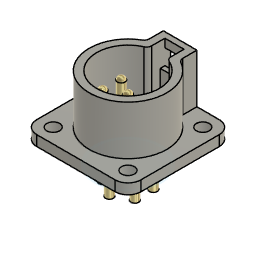
RPC1-12RB-6P_v13 (Autodesk Fusion 360 design; units mm, degrees)
Autodesk Fusion 360 part; units mm, degrees
sketch "Skizze1" plane through (0, 0, 0) normal (0, 0, 1) x (1, 0, 0)
  line L0 (-10.1, 10.1) -> (10.1, 10.1)
  line L1 (10.1, 10.1) -> (10.1, -10.1)
  line L2 (10.1, -10.1) -> (-10.1, -10.1)
  line L3 (-10.1, -10.1) -> (-10.1, 10.1)
  line L4 (0, 10.1) -> (0, -10.1) construction
  line L5 (-10.1, 0) -> (10.1, 0) construction
  line L6 (-7.25, 7.25) -> (7.25, 7.25) construction
  line L7 (7.25, 7.25) -> (7.25, -7.25) construction
  line L8 (7.25, -7.25) -> (-7.25, -7.25) construction
  line L9 (-7.25, -7.25) -> (-7.25, 7.25) construction
  circle A0 centre (0, 0) radius 7.5
  circle A1 centre (0, 0) radius 6.05
  line L10 (-3.25, 10.1) -> (3.25, 10.1)
  line L11 (3.25, 10.1) -> (3.25, 5.1029)
  line L12 (3.25, 5.1029) -> (-3.25, 5.1029)
  line L13 (-3.25, 5.1029) -> (-3.25, 10.1)
  line L14 (1.85, 8.7) -> (1.85, 6.5029)
  line L15 (1.85, 6.5029) -> (-1.85, 6.5029)
  line L16 (-1.85, 6.5029) -> (-1.85, 8.7)
  line L17 (-1.85, 8.7) -> (1.85, 8.7)
  line L18 (-1.85, 6.5029) -> (-1.85, 5.1029)
  line L19 (1.85, 6.5029) -> (1.85, 5.1029)
  circle A2 centre (0, -3.6) radius 0.76
  circle A3 centre (3.12, -1.8) radius 0.76
  circle A4 centre (3.12, 1.8) radius 0.76
  circle A5 centre (-3.12, 1.8) radius 0.76
  circle A6 centre (-3.12, -1.8) radius 0.76
  circle A7 centre (0, 0) radius 0.76
  line L20 (-1.85, 8.7) -> (1.85, 8.7)
  line L21 (1.85, 8.7) -> (1.85, 9)
  line L22 (1.85, 9) -> (-1.85, 9)
  line L23 (-1.85, 9) -> (-1.85, 8.7)
  line L24 (-1.85, 8.1) -> (1.85, 8.1)
  line L25 (3.12, -3.6) -> (-3.12, -3.6) construction
  line L26 (-3.12, -3.6) -> (-3.12, 1.8) construction
  line L27 (-3.12, 1.8) -> (3.12, 1.8) construction
  line L28 (3.12, 1.8) -> (3.12, -3.6) construction
  circle A8 centre (0, 0) radius 6.4
  dimension "d1" = 20.2
  dimension "d2" = 20.2
  dimension "d3" = 14.5
  dimension "d4" = 14.5
  dimension "d5" = 15
  dimension "d6" = 12.1
  dimension "d7" = 6.5
  dimension "d8" = 1.4
  dimension "d20" = 1.52
  dimension "d23" = 1.52
  dimension "d41" = 1.1
  dimension "d42" = 2
  dimension "d68" = 6.24
  dimension "d69" = 3.6
  dimension "d70" = 1.8
  dimension "d71" = 3.12
  dimension "d72" = 1.8
  dimension "d73" = 1.8
  dimension "d78" = 12.8
  constraint horizontal L0
  constraint vertical L1
  constraint horizontal L2
  constraint vertical L3
  constraint midpoint L0 L4.start
  constraint midpoint L2 L4.end
  constraint midpoint L3 L5.start
  constraint midpoint L1 L5.end
  constraint coincident A0.centre L5
  constraint coincident A0.centre L4
  constraint horizontal L6
  constraint vertical L7
  constraint horizontal L8
  constraint vertical L9
  constraint symmetric L4 L7 L9
  constraint symmetric L5 L6 L8
  constraint coincident A0.centre A1.centre
  constraint concentric A0 A1
  constraint horizontal L10
  constraint vertical L11
  constraint horizontal L12
  constraint vertical L13
  constraint coincident A1 L11.end
  constraint coincident L0 L10.start
  constraint symmetric L4 L11 L13
  constraint coincident L12 L18.end
  constraint perpendicular L12 L18
  constraint coincident L12 L19.end
  constraint perpendicular L12 L19
  constraint coincident L4 A2.centre
  constraint horizontal L20
  constraint vertical L21
  constraint horizontal L22
  constraint vertical L23
  constraint coincident L14.start L17.end
  constraint coincident L16 L24.start
  constraint coincident L14 L24.end
  constraint perpendicular L14 L24
  constraint horizontal L25
  constraint vertical L26
  constraint horizontal L27
  constraint vertical L28
  constraint coincident A4.centre L27.end
  constraint coincident A3.centre L28
  constraint coincident A6.centre L26
  constraint coincident A5.centre L26.end
  constraint coincident A2.centre L25
  measures "d1" distance of L1 L3
  measures "d2" distance of L0.end L1.end
  measures "d3" distance of L6 L8
  measures "d4" distance of L7 L9
  measures "d5" diameter of A0
  measures "d6" diameter of A1
  measures "d7" distance of L11 L13
  measures "d20" diameter of A2
  measures "d23" diameter of A7
  measures "d41" distance of L10 L22
  measures "d42" distance of L0 L24
  measures "d68" distance of A5.centre A4.centre
  measures "d69" distance of A0.centre L25
  measures "d70" vertical distance of A6.centre A0.centre
  measures "d71" distance of L4 A4.centre
  measures "d72" distance of L5 A3.centre
  measures "d73" distance of L5 A4.centre
  measures "d78" diameter of A8
extrude "Extrusion1" add sketch "Skizze1" against normal blind 2 contours L0 L1 L2 L3 A0 L11 L13 | L0 A0 L10 L11 L13 L14 L16 L21 L22 L23 | A0 L11 L13 A8 | A0 L13 L16 L18 A8 | A0 L11 L14 L19 A8 | A0 L14 L16 L24 | A0 L14 L15 L16 | A1 L13 L18 A8 | A1 L11 L13 A8 | A1 L11 L19 A8 | L15 L18 L19 A8 | L14 L16 L17 L20 L24 | A1 L12 | A1 L12 L18 | A1 L18 L19 A8 | A1 L12 L19 | L17 L20 L21 L22 L23 | A1 L12 L18 L19 | A2 | A3 | A4 | A5 | A6 | A7 makes body 1
extrude "Extrusion2" add sketch "Skizze1" against normal blind 6.2 contours A1 L13 L18 A8 | A1 L11 L13 A8 | A1 L11 L19 A8 | A1 L12 | A1 L12 L18 | A1 L18 L19 A8 | A1 L12 L19 | A1 L12 L18 L19 | A2 | A3 | A4 | A5 | A6 | A7 bodies 1
fillet "Abrundung1" radius 2.5 4 edges at (10.1, -10.1, -1) (-10.1, -10.1, -1) (-10.1, 10.1, -1) (10.1, 10.1, -1) on bodies 1
hole "Bohrung1" at (-7.25, -7.25, 0) at (-7.25, 7.25, 0) at (7.25, -7.25, 0) at (7.25, 7.25, 0) direction (0, 0, -1) diameter 2.5 end through all bodies 1
extrude "Extrusion3" add sketch "Skizze1" along normal blind 9.5 contours L0 A0 L10 L11 L13 L14 L16 L21 L22 L23 | A0 L11 L13 A8 | A0 L13 L16 L18 A8 | A0 L11 L14 L19 A8 | A1 L13 L18 A8 | A1 L11 L13 A8 | A1 L11 L19 A8 bodies 1
extrude "Extrusion4" [suppressed]
fillet "Abrundung2" [suppressed]
sketch "Skizze2" plane through (0, 10.1, 0) normal (0, 1, 0) x (-1, 0, 0)
  line L0 (-7.6, 0) -> (-7.6, -2)
  line L1 (-7.6, -2) -> (7.6, -2)
  line L2 (7.6, -2) -> (7.6, 0)
  line L3 (7.6, 0) -> (3.25, 0)
  line L4 (3.25, 0) -> (3.25, 9.5)
  line L5 (3.25, 9.5) -> (-3.25, 9.5)
  line L6 (-3.25, 9.5) -> (-3.25, 0)
  line L7 (-3.25, 0) -> (-7.6, 0)
  line L8 (-1.85, 7.9) -> (1.85, 7.9)
  line L9 (1.85, 0) -> (-1.85, 0)
  line L10 (-1.85, 0) -> (-1.85, 7.9)
  line L11 (-1.85, 0) -> (-1.85, 9.5)
  line L12 (1.85, 0) -> (1.85, 9.5)
  point P0 (1.85, 9.5)
  dimension "d28" = 1.6
  constraint horizontal L8
  constraint horizontal L9
  constraint vertical L10
  constraint coincident L8.start L11
  constraint coincident L9.end L10.start
  constraint coincident P0 L12.end
  constraint perpendicular L5 L12
  constraint coincident L8.end L12
  measures "d28" distance of L5 L8
extrude "Extrusion5" cut sketch "Skizze2" against normal up to surface (1.1 mm away) contours L8 L9 L10 L11 L12 bodies 1
sketch "Skizze1 (2)" plane through (0, 0, 9.5) normal (0, 0, 1) x (-1, 0, 0) in component "cable:end"
  line L0 (1.85, -5.7602) -> (1.85, -9)
  line L1 (-1.85, -9) -> (-1.85, -5.7602)
  arc A0 (1.85, -5.7602) -> (-1.85, -5.7602) centre (0, 0) ccw
  line L2 (3.25, -10.1) -> (3.25, -6.7593)
  arc A1 (3.25, -6.7593) -> (-3.25, -6.7593) centre (0, 0) ccw
  line L3 (-3.25, -6.7593) -> (-3.25, -10.1)
  line L4 (-3.25, -10.1) -> (3.25, -10.1)
  circle A2 centre (3.0311, -1.75) radius 0.75
  circle A3 centre (3.0311, 1.75) radius 0.75
  circle A4 centre (0, 3.5) radius 0.75
  circle A5 centre (-3.0311, 1.75) radius 0.75
  circle A6 centre (-3.0311, -1.75) radius 0.75
  circle A7 centre (0, 0) radius 0.75
  circle A8 centre (0, 0) radius 7.5
  line L5 (1.85, -9) -> (-1.85, -9)
  constraint concentric A7 A8
  constraint coincident A1.end A8
extrude "Extrusion1'" [suppressed] in component "cable:end"
ref_plane "Arbeitsebene1" through (0, 1.3, 40.5) normal (0, 0, 1) x (-1, 0, 0) in component "cable:end"
sketch "Skizze2 (2)" plane through (0, 0, 40.5) normal (0, 0, 1) x (1, 0, 0) in component "cable:end"
  circle A0 centre (0, 0) radius 6.05
  circle A1 centre (0.1335, 0.0008) radius 7.4424
  point P0 (1.85, 5.7602)
  point P1 (3.25, 6.7593)
  constraint coincident A0.centre origin
  constraint coincident A0 P0
  constraint coincident A1 P1
loft "Erhebung1" [suppressed] in component "cable:end"
sketch "Skizze3" plane through (0, 10.1, 0) normal (0, 1, 0) x (-1, 0, 0) in component "cable:end"
  line L0 (-1.85, 0) -> (-1.85, 7.9)
  line L1 (-1.85, 7.9) -> (1.85, 7.9)
  line L2 (1.85, 7.9) -> (1.85, 0)
  line L3 (1.85, 0) -> (-1.85, 0)
  line L4 (-7.6, 0) -> (-7.6, -2)
  line L5 (-7.6, -2) -> (7.6, -2)
  line L6 (7.6, -2) -> (7.6, 0)
  line L7 (7.6, 0) -> (3.25, 0)
  line L8 (3.25, 0) -> (3.25, 9.5)
  line L9 (3.25, 9.5) -> (-3.25, 9.5)
  line L10 (-3.25, 9.5) -> (-3.25, 0)
  line L11 (-3.25, 0) -> (-7.6, 0)
  line L12 (-3.25, 9.5) -> (3.25, 9.5)
  line L13 (3.25, 9.5) -> (3.25, 16.5)
  line L14 (3.25, 16.5) -> (-3.25, 16.5)
  line L15 (-3.25, 16.5) -> (-3.25, 9.5)
  dimension "d34" = 7
  constraint horizontal L12
  constraint vertical L13
  constraint horizontal L14
  constraint vertical L15
  constraint coincident L9.end L10.start
  constraint coincident L8.end L9.start
  measures "d34" distance of L12 L14
extrude "Extrusion2'" [suppressed] in component "cable:end"
sketch "Skizze4" plane through (0, 10.1, 0) normal (0, 1, 0) x (-1, 0, 0) in component "cable:end"
  line L0 (-1.7301, 14.2327) -> (1.7301, 14.2327)
  line L1 (1.7301, 14.2327) -> (1.7301, 11)
  line L2 (1.7301, 11) -> (-1.7301, 11)
  line L3 (-1.7301, 11) -> (-1.7301, 14.2327)
  line L4 (3.25, 16.5) -> (-3.25, 16.5)
  line L5 (7.5, 9.5) -> (-7.5, 9.5)
  line L6 (0, 16.5) -> (0, 9.5)
  line L7 (3.25, 16.5) -> (-3.25, 16.5)
  constraint horizontal L0
  constraint vertical L1
  constraint horizontal L2
  constraint vertical L3
  constraint midpoint L4 L6.start
  constraint coincident L5 L6.end
  constraint perpendicular L6 L7
  constraint symmetric L1 L3 L6
extrude "Extrusion3'" [suppressed] in component "cable:end"
fillet "Abrundung1'" [suppressed] in component "cable:end"
sketch "Skizze3 (2)" plane through (0, 0, 0) normal (0, 0, 1) x (-1, 0, 0)
  arc A0 (1.85, -5.7602) -> (-1.85, -5.7602) centre (0, 0) ccw
  line L0 (-1.85, -5.7602) -> (-1.85, -10.1)
  line L1 (-1.85, -10.1) -> (1.85, -10.1)
  line L2 (1.85, -10.1) -> (1.85, -5.7602)
  line L3 (1.85, -8.7) -> (-1.85, -8.7)
  line L4 (-1.85, -8.7) -> (-1.85, -7.9301)
  line L5 (-1.85, -7.9301) -> (1.85, -7.9301)
  line L6 (1.85, -7.9301) -> (1.85, -8.7)
  point P0 (1.85, -5.7602)
  point P1 (1.85, -9)
  constraint horizontal L3
  constraint vertical L4
  constraint horizontal L5
  constraint vertical L6
  constraint midpoint L0 L4.end
extrude "Extrusion6" add sketch "Skizze1" along normal up to surface (4.9 mm away) contours L14 L16 L17 L20 L24 | L17 L20 L21 L22 L23 bodies 1
extrude "Extrusion7" cut sketch "Skizze1" against normal up to surface (6.2 mm away) contours A2 | A3 | A4 | A5 | A6 | A7 bodies 1
sketch "Skizze1 (3)" plane through (0, 0, 0) normal (0, 1, 0) x (1, 0, 0) in component "pin"
  line L0 (0, 9.75) -> (0, -6.25)
  line L1 (0, -6.25) -> (-0.76, -6.25)
  line L2 (-0.76, -6.25) -> (-0.76, 9.7726)
  line L3 (-0.76, 9.7726) -> (0, 9.75)
  circle A0 centre (0, -5.49) radius 0.76
  line L4 (6.05, -9.5) -> (-6.05, -9.5)
  dimension "d47" = 16
  dimension "d48" = 0.76
  dimension "d49" = 3.25
  constraint vertical L0
  constraint perpendicular L0 L1
  constraint perpendicular L1 L2
  constraint coincident L0 A0.centre
  constraint tangent L2 A0
  constraint tangent L1 A0
  measures "d47" distance of L0.start L0.end
  measures "d48" distance of L0 L2
  measures "d49" distance of L1 L4
revolve "Drehen1" add sketch "Skizze1 (3)" angle 360 about axis through (0, 0, -9.75) along (0, 0, 1) separate body contours L0 L2 L3 A0 | L0 A0 picked at (-0.4219, -5.2973) makes body 3 in component "pin"
sketch "Skizze4 (2)" plane through (0, 0, -6.2) normal (0, 0, -1) x (1, 0, 0)
  circle A0 centre (0, 3.6) radius 0.76
  circle A1 centre (-3.12, -1.8) radius 0.76
  circle A2 centre (3.12, 1.8) radius 0.76
  circle A3 centre (0, 0) radius 0.76
  circle A4 centre (-3.12, 1.8) radius 0.76
  circle A5 centre (3.12, -1.8) radius 0.76
  circle A6 centre (0, 0) radius 6.05
  circle A7 centre (0, -3.8) radius 0.6
  line L0 (0, -10.1) -> (0, 10.1)
  circle A8 centre (0, 0) radius 6.4
  dimension "d51" = 12.1
  dimension "d56" = 3.8
  dimension "d57" = 1.2
  constraint concentric A3 A6
  constraint coincident A7.centre L0
  measures "d51" diameter of A6
  measures "d56" distance of A3.centre A7.centre
  measures "d57" diameter of A7
extrude "Extrusion8" cut sketch "Skizze4 (2)" against normal blind 1.6 contours A0 A3 A6 A7 L0 | A0 A3 A6 A7 L0 | A7 L0 | A7 L0 bodies 1
extrude "Extrusion1''" [no effect] in component "pin"
extrude "Extrusion9" cut sketch "Skizze4 (2)" against normal up to surface (5.6 mm away) contours A7 L0 | A7 L0 bodies 1
fillet "Abrundung3" radius 1 2 edges at (3.25, 6.7593, 4.75) (-3.25, 6.7593, 4.75) on bodies 1
fillet "Abrundung4" radius 1 2 edges at (-1.85, 5.7602, 4.75) (1.85, 5.7602, 4.75) on bodies 1
pattern_linear "00000000-0000-0000-0000-000000000000" [suppressed]
sketch "Skizze1 (4)" plane through (0, 0, -4.6) normal (0, 0, -1) x (1, 0, 0) in component "pcb"
  circle A0 centre (0, -3.8) radius 0.6
  circle A1 centre (3.12, 1.8) radius 0.76
  circle A2 centre (-3.12, 1.8) radius 0.76
  circle A3 centre (0, 0) radius 0.76
  circle A4 centre (-3.12, -1.8) radius 0.76
  circle A5 centre (0, 3.6) radius 0.76
  circle A6 centre (3.12, -1.8) radius 0.76
  circle A7 centre (0, 0) radius 6.05
  circle A8 centre (0, -3.8) radius 0.8
  circle A9 centre (0, 0) radius 5.95
  dimension "d74" = 0.2
  dimension "d75" = -0.1
extrude "Extrusion1'''" add sketch "Skizze1 (4)" along normal up to surface (1.6 mm away) separate body contours A9 makes body 4 in component "pcb"
sketch "Skizze5" plane through (0, 0, -6.2) normal (0, 0, -1) x (1, 0, 0)
  circle A0 centre (0, 0) radius 6.05
  circle A1 centre (0, 0) radius 6.4
extrude "Extrusion10" cut sketch "Skizze5" against normal up to surface (4.2 mm away) bodies 1
component "pin" placed x (1, 0, 0) y (0, 1, 0) z (0, 0, 1) at (0, 0, 0)
component "pcb" placed x (1, 0, 0) y (0, 1, 0) z (0, 0, 1) at (0, 0, 0)
component "pin" placed x (1, 0, 0) y (0, 1, 0) z (0, 0, 1) at (3.12, -1.8, 0)
component "pin" placed x (1, 0, 0) y (0, 1, 0) z (0, 0, 1) at (-3.12, -1.8, 0)
component "pin" placed x (1, 0, 0) y (0, 1, 0) z (0, 0, 1) at (3.12, 1.8, 0)
component "pin" placed x (1, 0, 0) y (0, 1, 0) z (0, 0, 1) at (-3.12, 1.8, 0)
component "pin" placed x (1, 0, 0) y (0, 1, 0) z (0, 0, 1) at (0, -3.6, 0)
equation "d11 = -4.2 mm - 2 mm"
equation "d20 = d23"
equation "d48 = ( 1.52 / 2 ) * 1 mm"
equation "d68 = ( 3.12 * 2 ) * 1 mm"
